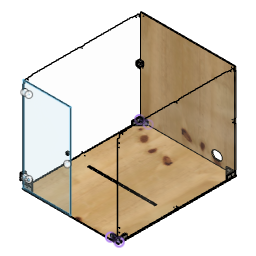
Prusa Mk3 Case (Autodesk Fusion 360 design; units mm, degrees)
Autodesk Fusion 360 part; units mm, degrees
note: some values were not read from the file. Set by a fixed rule: which sketch regions a step uses.
sketch "Sketch1" plane through (0, 0, 0) normal (0, 0, 1) x (1, 0, 0) in component "winkel"
  line L0 (0, 0) -> (42.4, 0)
  line L1 (42.4, 0) -> (42.4, 40)
  line L2 (42.4, 40) -> (0, 40)
  line L3 (0, 40) -> (0, 0)
  line L4 (2, 0) -> (2, 40)
  line L5 (4.4, 40) -> (4.4, 0)
  line L6 (7.4, 0) -> (7.4, 35)
  line L7 (7.4, 35) -> (42.4, 35)
  circle A0 centre (17.8289, 24.5711) radius 2
  line L8 (7.4, 5.6569) -> (36.7431, 35)
  line L9 (7.4, 0) -> (42.4, 35)
  line L10 (18.0066, 16.2635) -> (20.835, 13.435)
  line L11 (26.1365, 24.3934) -> (28.965, 21.565)
  line L12 (4.4, 35) -> (2, 35)
  line L13 (7.4, 35) -> (22.0716, 20.3284)
  dimension "d1" = 2.4
  dimension "d4" = 2
  dimension "d6" = 3
  dimension "d14" = 4
  dimension "d17" = 4
  dimension "d19" = 15
  dimension "d20" = 15
  dimension "d73" = 5
  dimension "d74" = 5
  dimension "d238" = 35
  dimension "d239" = 35
  dimension "d240" = 6
  constraint horizontal L0
  constraint vertical L1
  constraint horizontal L2
  constraint vertical L3
  constraint coincident L0.start L3.end
  constraint coincident L0 L4.start
  constraint perpendicular L0 L4
  constraint coincident L0 L6.start
  constraint perpendicular L0 L6
  constraint coincident L1 L7.end
  constraint perpendicular L1 L7
  constraint coincident L6 L8.start
  constraint coincident L7 L8.end
  constraint coincident L8 L10.start
  constraint coincident L9 L10.end
  constraint perpendicular L9 L10
  constraint coincident L8 L11.start
  constraint coincident L9 L11.end
  constraint perpendicular L9 L11
  constraint parallel L8 L9
  constraint coincident L2 L4.end
  constraint coincident L2 L5.start
  constraint coincident L5 L12.start
  constraint coincident L4 L12.end
  constraint perpendicular L4 L12
  constraint midpoint L8 L13.end
  constraint coincident A0.centre L13
  measures "d1" distance of L4 L5
  measures "d4" distance of L3 L4
  measures "d6" distance of L5 L6
  measures "d14" diameter of A0
  measures "d17" distance of L8 L9
  measures "d19" distance of L8.start L10
  measures "d20" distance of L8.end L11
  measures "d73" distance of L2 L7
  measures "d74" distance of L2 L12
  measures "d238" distance of L1 L6
  measures "d239" distance of L0 L7
  measures "d240" distance of A0.centre L8
extrude "Extrude1" add sketch "Sketch1" against normal blind 3 contours L0 L2 L3 L4 | L0 L4 L5 L12 | L0 L1 L2 L5 L6 L7 | L2 L4 L5 L12 | L6 L8 L9 L10 | L6 A0 L8 L13 | L8 L9 L10 L11 | L7 L8 L9 L11 | L7 A0 L8 L13 makes body 1 in component "winkel"
extrude "Extrude2" add sketch "Sketch1" along normal blind 15 contours L0 L2 L3 L4 | L0 L1 L2 L5 L6 L7 | L2 L4 L5 L12 | L6 L8 L9 L10 | L7 L8 L9 L11 bodies 1 in component "winkel"
extrude "Extrude3" add sketch "Sketch1" along normal blind 15 contours L6 L8 L9 L10 | L7 L8 L9 L11 bodies 1 in component "winkel"
chamfer "Chamfer1" distance 13 distance2 14 2 edges at (19.4208, 14.8492, 15) (27.5508, 22.9792, 15) measured on face at (26.381, 38.3333, 15) measured on face at (26.381, 38.3333, 15) on bodies 1 in component "winkel"
sketch "Sketch2" plane through (0, 40, 0) normal (0, 1, 0) x (-1, 0, 0) in component "winkel"
  line L0 (-42.4, 15) -> (-42.4, -3)
  line L1 (-42.4, -3) -> (0, -3)
  line L2 (0, -3) -> (0, 15)
  line L3 (0, 15) -> (-42.4, 15)
  circle A0 centre (-20, 7) radius 1.75
  line L4 (0, 0) -> (-42.4, 0)
  dimension "d119" = 20
  dimension "d120" = 7
  dimension "d267" = 3.5
  measures "d119" distance of L2 A0.centre
  measures "d120" distance of A0.centre L4
  measures "d267" diameter of A0
extrude "Extrude4" cut sketch "Sketch2" against normal blind 13 contours A0 bodies 1 in component "winkel"
sketch "Sketch3" plane through (0, 0, 0) normal (-1, 0, 0) x (0, -1, 0) in component "winkel"
  line L0 (-40, 15) -> (-40, -3)
  line L1 (-40, -3) -> (0, -3)
  line L2 (0, -3) -> (0, 15)
  line L3 (0, 15) -> (-40, 15)
  circle A0 centre (-20, 7) radius 1.75
  line L4 (-40, 8.75) -> (-40, 5.25)
  dimension "d264" = 20
  dimension "d265" = 7
  dimension "d266" = 3.5
  measures "d264" distance of A0.centre L4
  measures "d265" vertical distance of origin A0.centre
  measures "d266" diameter of A0
extrude "Extrude5" cut sketch "Sketch3" against normal blind 20 contours A0 bodies 1 in component "winkel"
mirror "MirrorComponent2" about plane through (0, 0, 0) normal (0, 0, 1) of bodies 1 makes body 2 in component "winkel(Mirror)"
sketch "Sketch1 (2)" plane through (0, 0, 0) normal (0, 0, 1) x (1, 0, 0) in component "grundplatte"
  line L0 (0, 0) -> (470, 0)
  line L1 (470, 0) -> (470, -580)
  line L2 (470, -580) -> (0, -580)
  line L3 (0, -580) -> (0, 0)
  circle A0 centre (18, -20) radius 1.75
  circle A1 centre (452, -20) radius 1.75
  circle A2 centre (18, -560) radius 1.75
  circle A3 centre (452, -560) radius 1.75
  circle A4 centre (16, -290) radius 1.75
  circle A5 centre (454, -290) radius 1.75
  line L4 (70, -320) -> (400, -320)
  line L5 (400, -320) -> (400, -330)
  line L6 (400, -330) -> (70, -330)
  line L7 (70, -330) -> (70, -320)
  dimension "d27" = 580
  dimension "d28" = 470
  dimension "d31" = 18
  dimension "d32" = 20
  dimension "d252" = 3.5
  dimension "d253" = 18
  dimension "d254" = 20
  dimension "d255" = 16
  dimension "d256" = 16
  dimension "d309" = 290
  dimension "d358" = 330
  dimension "d359" = 10
  dimension "d360" = 250
  dimension "d361" = 70
  constraint horizontal L0
  constraint vertical L1
  constraint horizontal L2
  constraint vertical L3
  constraint coincident L0.start L3.end
  constraint equal A0 A1
  constraint horizontal A0.centre A1.centre
  constraint equal A2 A3
  constraint equal A1 A3
  constraint vertical A1.centre A3.centre
  constraint horizontal A2.centre A3.centre
  constraint vertical A0.centre A2.centre
  constraint equal A4 A5
  constraint equal A2 A4
  constraint horizontal A4.centre A5.centre
  constraint horizontal L4
  constraint vertical L5
  constraint horizontal L6
  constraint vertical L7
  measures "d27" distance of L0.start L2.end
  measures "d28" distance of L1.end L2.end
  measures "d31" distance of L3 A0.centre
  measures "d32" distance of L0 A0.centre
  measures "d252" diameter of A0
  measures "d253" distance of L1 A1.centre
  measures "d254" distance of L2 A2.centre
  measures "d255" distance of L3 A4.centre
  measures "d256" distance of L1 A5.centre
  measures "d309" distance of L2 A4.centre
  measures "d358" distance of L5.end L6.end
  measures "d359" distance of L4.start L6.end
  measures "d360" distance of L2 L6
  measures "d361" distance of L3 L6.end
extrude "Extrude1'" add sketch "Sketch1 (2)" along normal blind 5 separate body makes body 3 in component "grundplatte"
sketch "Sketch1 (3)" plane through (0, 0, 0) normal (1, 0, 0) x (0, 1, 0) in component "seite"
  line L0 (179.5, 146.2971) -> (-400.5, 146.2971)
  line L1 (-400.5, 146.2971) -> (-400.5, 606.2971)
  line L2 (-400.5, 606.2971) -> (179.5, 606.2971)
  line L3 (179.5, 606.2971) -> (179.5, 146.2971)
  line L4 (179.5, 149.5971) -> (134.5, 149.5971)
  line L5 (134.5, 149.5971) -> (134.5, 146.2971)
  line L6 (-400.5, 149.5971) -> (-355.5, 149.5971)
  line L7 (-355.5, 149.5971) -> (-355.5, 146.2971)
  line L8 (-400.5, 164.2971) -> (-390.5, 164.2971)
  line L9 (-390.5, 164.2971) -> (-390.5, 149.5971)
  line L10 (179.5, 164.2971) -> (169.5, 164.2971)
  line L11 (169.5, 164.2971) -> (169.5, 146.2971)
  line L12 (-400.5, 588.2971) -> (-390.5, 588.2971)
  line L13 (-390.5, 588.2971) -> (-390.5, 602.9971)
  line L14 (-390.5, 602.9971) -> (-355.5, 602.9971)
  line L15 (-355.5, 602.9971) -> (-355.5, 606.2971)
  line L16 (134.5, 606.2971) -> (134.5, 602.9971)
  line L17 (134.5, 602.9971) -> (169.5, 602.9971)
  line L18 (169.5, 602.9971) -> (169.5, 588.2971)
  line L19 (169.5, 588.2971) -> (179.5, 588.2971)
  circle A0 centre (170.5, 206.2971) radius 1.75
  circle A1 centre (170.5, 186.2971) radius 1.75
  circle A2 centre (170.5, 566.2971) radius 1.75
  circle A3 centre (170.5, 546.2971) radius 1.75
  line L20 (-100, 146.2971) -> (-100, 149.5971)
  line L21 (-100, 149.5971) -> (-121, 149.5971)
  line L22 (-121, 149.5971) -> (-121, 146.2971)
  line L23 (-100, 606.2971) -> (-100, 602.9971)
  line L24 (-100, 602.9971) -> (-121, 602.9971)
  line L25 (-121, 602.9971) -> (-121, 606.2971)
  line L26 (-400.5, 386.7971) -> (-392.2, 386.7971)
  line L27 (-392.2, 386.7971) -> (-392.2, 365.7971)
  line L28 (-392.2, 365.7971) -> (-400.5, 365.7971)
  circle A4 centre (154.5, 156.2971) radius 1.75
  circle A5 centre (154.5, 596.2971) radius 1.75
  circle A6 centre (-375.5, 596.2971) radius 1.75
  circle A7 centre (-375.5, 156.2971) radius 1.75
  circle A8 centre (-385.2, 376.2971) radius 1.75
  circle A9 centre (-110.5, 156.5971) radius 1.75
  circle A10 centre (-110.5, 595.9971) radius 1.75
  dimension "d33" = 580
  dimension "d44" = 3.3
  dimension "d45" = 45
  dimension "d46" = 45
  dimension "d47" = 3.3
  dimension "d77" = 18
  dimension "d78" = 10
  dimension "d79" = 18
  dimension "d80" = 10
  dimension "d90" = 460
  dimension "d91" = 10
  dimension "d92" = 10
  dimension "d93" = 18
  dimension "d94" = 18
  dimension "d95" = 3.3
  dimension "d96" = 3.3
  dimension "d97" = 45
  dimension "d98" = 45
  dimension "d197" = 20
  dimension "d198" = 3.5
  dimension "d200" = 40
  dimension "d201" = 9
  dimension "d205" = 20
  dimension "d206" = 40
  dimension "d231" = 21
  dimension "d232" = 3.3
  dimension "d233" = 279.5
  dimension "d234" = 3.3
  dimension "d257" = 21
  dimension "d258" = 8.3
  dimension "d259" = 219.5
  dimension "d270" = 25
  dimension "d271" = 25
  dimension "d272" = 3.5
  dimension "d273" = 10
  dimension "d274" = 10
  dimension "d280" = 10.5
  dimension "d281" = 3.5
  dimension "d282" = 7
  dimension "d283" = 3.5
  dimension "d284" = 10.5
  dimension "d285" = 7
  dimension "d286" = 3.5
  dimension "d287" = 10.5
  dimension "d288" = 7
  constraint horizontal L0
  constraint vertical L1
  constraint horizontal L2
  constraint vertical L3
  constraint coincident L3 L4.start
  constraint perpendicular L3 L4
  constraint coincident L0 L5.end
  constraint perpendicular L0 L5
  constraint coincident L1 L6.start
  constraint perpendicular L1 L6
  constraint coincident L0 L7.end
  constraint perpendicular L0 L7
  constraint coincident L1 L8.start
  constraint perpendicular L1 L8
  constraint coincident L6 L9.end
  constraint perpendicular L6 L9
  constraint coincident L3 L10.start
  constraint perpendicular L3 L10
  constraint coincident L0 L11.end
  constraint perpendicular L0 L11
  constraint coincident L1 L12.start
  constraint perpendicular L1 L12
  constraint perpendicular L12 L13
  constraint perpendicular L13 L14
  constraint coincident L2 L15.end
  constraint perpendicular L2 L15
  constraint coincident L2 L16.start
  constraint perpendicular L2 L16
  constraint perpendicular L16 L17
  constraint perpendicular L17 L18
  constraint coincident L3 L19.end
  constraint perpendicular L3 L19
  constraint equal A0 A1
  constraint vertical A0.centre A1.centre
  constraint equal A2 A3
  constraint equal A0 A3
  constraint vertical A0.centre A3.centre
  constraint coincident L0 L20.start
  constraint perpendicular L0 L20
  constraint perpendicular L20 L21
  constraint coincident L0 L22.end
  constraint perpendicular L21 L22
  constraint coincident L2 L23.start
  constraint perpendicular L2 L23
  constraint perpendicular L23 L24
  constraint coincident L2 L25.end
  constraint perpendicular L2 L25
  constraint vertical L20.end L23.end
  constraint vertical L21.end L24.end
  constraint coincident L1 L26.start
  constraint perpendicular L1 L26
  constraint perpendicular L26 L27
  constraint perpendicular L27 L28
  constraint horizontal A5.centre A6.centre
  constraint vertical A6.centre A7.centre
  constraint horizontal A4.centre A7.centre
  constraint vertical A4.centre A5.centre
  constraint equal A5 A6
  constraint equal A6 A7
  constraint equal A4 A7
  measures "d33" distance of L1.end L2.end
  measures "d44" distance of L4.end L5.end
  measures "d45" distance of L4.start L4.end
  measures "d46" distance of L6.start L6.end
  measures "d47" distance of L6.end L7.end
  measures "d77" distance of L0 L8
  measures "d78" distance of L8.start L8.end
  measures "d79" distance of L0 L10
  measures "d80" distance of L10.start L10.end
  measures "d90" distance of L0.end L1.end
  measures "d91" distance of L18.end L19.end
  measures "d92" distance of L12.start L12.end
  measures "d93" distance of L2 L12.end
  measures "d94" distance of L2 L18.end
  measures "d95" distance of L16.start L16.end
  measures "d96" distance of L14.end L15.end
  measures "d97" distance of L1 L14.end
  measures "d98" distance of L3 L16.end
  measures "d197" distance of A0.centre A1.centre
  measures "d198" diameter of A0
  measures "d200" distance of L0 A1.centre
  measures "d201" distance of L3 A0.centre
  measures "d205" distance of A2.centre A3.centre
  measures "d206" distance of L2 A2.centre
  measures "d231" distance of L20.end L21.end
  measures "d232" distance of L20.start L20.end
  measures "d233" distance of L3 L20
  measures "d234" distance of L23.start L23.end
  measures "d257" distance of L26.end L27.end
  measures "d258" distance of L26.start L26.end
  measures "d259" distance of L0 L27.end
  measures "d270" distance of L3 A5.centre
  measures "d271" distance of L1 A6.centre
  measures "d272" diameter of A5
  measures "d273" distance of L2 A5.centre
  measures "d274" distance of L0 A4.centre
  measures "d280" distance of L28 A8.centre
  measures "d281" diameter of A8
  measures "d282" distance of L27 A8.centre
  measures "d283" diameter of A9
  measures "d284" distance of L22 A9.centre
  measures "d285" distance of L21 A9.centre
  measures "d286" diameter of A10
  measures "d287" distance of L25 A10.centre
  measures "d288" distance of L24 A10.centre
extrude "Extrude1''" add sketch "Sketch1 (3)" along normal blind 2 separate body contours L0 L1 L2 L3 L4 L5 L6 L7 L8 L9 L10 L11 L12 L13 L14 L15 L16 L17 L18 L19 L20 L21 L22 L23 L24 L25 L26 L27 L28 makes body 4 in component "seite"
sketch "Sketch1 (4)" plane through (0, 0, 0) normal (0, 1, 0) x (1, 0, 0) in component "hinten"
  line L0 (10.4, -408.1183) -> (471, -408.1183)
  line L1 (471, -408.1183) -> (471, 51.8817)
  line L2 (471, 51.8817) -> (10.4, 51.8817)
  line L3 (10.4, 51.8817) -> (10.4, -408.1183)
  circle A0 centre (456, 41.8817) radius 1.75
  circle A1 centre (25.4, 41.8817) radius 1.75
  circle A2 centre (456, -398.1183) radius 1.75
  circle A3 centre (25.4, -398.1183) radius 1.75
  line L4 (379, -8.1183) -> (391, -8.1183)
  arc A4 (391, -8.1183) -> (391, 31.8817) centre (391, 11.8817) ccw
  line L5 (391, 31.8817) -> (379, 31.8817)
  arc A5 (379, 31.8817) -> (379, -8.1183) centre (379, 11.8817) ccw
  line L6 (359, 11.8817) -> (411, 11.8817) construction
  circle A6 centre (21.4, -178.1183) radius 1.75
  circle A7 centre (460, -178.1183) radius 1.75
  dimension "d121" = 460
  dimension "d122" = 460.6
  dimension "d129" = 3.5
  dimension "d130" = 10
  dimension "d131" = 10
  dimension "d132" = 15
  dimension "d133" = 15
  dimension "d242" = 20
  dimension "d243" = 12
  dimension "d260" = 3.5
  dimension "d261" = 230
  dimension "d262" = 11
  dimension "d263" = 11
  dimension "d356" = 80
  dimension "d357" = 40
  constraint horizontal L0
  constraint vertical L1
  constraint horizontal L2
  constraint vertical L3
  constraint equal A1 A3
  constraint equal A0 A2
  constraint equal A2 A3
  constraint horizontal A2.centre A3.centre
  constraint vertical A0.centre A2.centre
  constraint horizontal A0.centre A1.centre
  constraint vertical A1.centre A3.centre
  constraint tangent L4 A4
  constraint tangent A4 L5
  constraint parallel L4 L5
  constraint tangent L5 A5
  constraint tangent L4 A5
  constraint midpoint A5 L6.start
  constraint midpoint A4 L6.end
  constraint horizontal L6
  constraint equal A6 A7
  constraint horizontal A6.centre A7.centre
  measures "d121" distance of L0.start L2.end
  measures "d122" distance of L0.start L0.end
  measures "d129" diameter of A3
  measures "d130" distance of L0 A2.centre
  measures "d131" distance of L2 A0.centre
  measures "d132" distance of L1 A0.centre
  measures "d133" distance of L3 A3.centre
  measures "d242" radius of A4
  measures "d243" distance of L4.start L4.end
  measures "d260" diameter of A7
  measures "d261" distance of L2 A6.centre
  measures "d262" distance of L3 A6.centre
  measures "d263" distance of L1 A7.centre
  measures "d356" distance of L1 A4.centre
  measures "d357" distance of L2 A5.centre
extrude "Extrude1'''" add sketch "Sketch1 (4)" along normal blind 5 separate body makes body 5 in component "hinten"
sketch "Sketch1 (5)" plane through (0, 0, 0) normal (0, 0, 1) x (1, 0, 0) in component "scharnier_1"
  line L0 (-72.6357, -505.4656) -> (-64.6357, -505.4656)
  line L1 (-64.6357, -505.4656) -> (-64.6357, -480.4656)
  line L2 (-64.6357, -480.4656) -> (-72.6357, -480.4656)
  line L3 (-72.6357, -480.4656) -> (-72.6357, -505.4656)
  circle A0 centre (-68.6357, -501.4656) radius 1.5
  line L4 (-72.6357, -495.4656) -> (-64.6357, -495.4656)
  dimension "d136" = 25
  dimension "d137" = 8
  dimension "d138" = 3
  dimension "d139" = 4
  dimension "d140" = 4
  dimension "d141" = 10
  constraint horizontal L0
  constraint vertical L1
  constraint horizontal L2
  constraint vertical L3
  constraint coincident L3 L4.start
  constraint coincident L1 L4.end
  constraint perpendicular L1 L4
  measures "d136" distance of L0.start L2.end
  measures "d137" distance of L1.end L2.end
  measures "d138" diameter of A0
  measures "d139" distance of L3 A0.centre
  measures "d140" distance of L0 A0.centre
  measures "d141" distance of L0 L4
extrude "Extrude1''''" add sketch "Sketch1 (5)" along normal blind 30 separate body makes body 6 in component "scharnier_1"
extrude "Extrude2'" cut sketch "Sketch1 (5)" along normal blind 20 and the other way blind -10 contours L0 L1 L3 L4 bodies 6 in component "scharnier_1"
sketch "Sketch2 (2)" plane through (-64.6357, 0, 0) normal (1, 0, 0) x (0, 1, 0) in component "scharnier_1"
  line L0 (-505.4656, 20) -> (-495.4656, 20)
  line L1 (-495.4656, 20) -> (-495.4656, 10)
  line L2 (-495.4656, 10) -> (-505.4656, 10)
  line L3 (-505.4656, 10) -> (-505.4656, 0)
  line L4 (-505.4656, 0) -> (-480.4656, 0)
  line L5 (-480.4656, 0) -> (-480.4656, 30)
  line L6 (-480.4656, 30) -> (-505.4656, 30)
  line L7 (-505.4656, 30) -> (-505.4656, 20)
  circle A0 centre (-488.4656, 5) radius 1.75
  circle A1 centre (-488.4656, 25) radius 1.75
  circle A2 centre (-488.4656, 25) radius 3
  circle A3 centre (-488.4656, 5) radius 3
  dimension "d180" = 3.5
  dimension "d202" = 8
  dimension "d203" = 5
  dimension "d204" = 20
  dimension "d213" = 6
  constraint equal A0 A1
  constraint vertical A0.centre A1.centre
  constraint concentric A1 A2
  constraint concentric A0 A3
  constraint equal A2 A3
  measures "d180" diameter of A1
  measures "d202" distance of L5 A1.centre
  measures "d203" distance of L6 A1.centre
  measures "d204" distance of A0.centre A1.centre
  measures "d213" diameter of A3
extrude "Extrude3'" cut sketch "Sketch2 (2)" against normal blind 30 contours A0 | A1 bodies 6 in component "scharnier_1"
fillet "Fillet1" radius 3 5 edges at (-64.6357, -505.4656, 25) (-64.6357, -505.4656, 5) (-72.6357, -505.4656, 5) (-72.6357, -505.4656, 25) (-72.6357, -495.4656, 15) on bodies 6 in component "scharnier_1"
chamfer "Chamfer1'" distance 6 distance2 12.5 1 edges at (-72.6357, -480.4656, 15) measured on face at (-67.3024, -480.4656, 10) on bodies 6 in component "scharnier_1"
extrude "Extrude4'" cut sketch "Sketch2 (2)" along normal blind -4 and the other way blind 8 contours A2 | A3 bodies 6 in component "scharnier_1"
sketch "Sketch1 (6)" plane through (0, 0, 0) normal (0, 0, 1) x (1, 0, 0) in component "scharnier_2"
  line L0 (36, -516) -> (36, -526)
  line L1 (36, -526) -> (-4, -526)
  line L2 (-4, -526) -> (-4, -518)
  circle A0 centre (0, -522) radius 1.5
  line L3 (8, -516) -> (36, -516)
  line L4 (3, -518) -> (3, -519)
  line L5 (3, -519) -> (8, -519)
  line L6 (36, -521) -> (2.8865, -526)
  line L7 (8, -519) -> (8, -516)
  line L8 (-4, -518) -> (3, -518)
  dimension "d154" = 8
  dimension "d155" = 4
  dimension "d156" = 4
  dimension "d158" = 3
  dimension "d159" = 2
  dimension "d181" = 7
  dimension "d182" = 1
  dimension "d183" = 40
  dimension "d184" = 5
  constraint horizontal L8
  constraint vertical L0
  constraint horizontal L1
  constraint vertical L2
  constraint perpendicular L4 L8
  constraint perpendicular L4 L5
  constraint midpoint L0 L6.start
  constraint coincident L1 L6.end
  constraint vertical L7
  measures "d154" distance of L2.end L1.end
  measures "d155" distance of L1 A0.centre
  measures "d156" distance of L2 A0.centre
  measures "d158" diameter of A0
  measures "d159" distance of L3 L8
  measures "d181" distance of L2.end L4.start
  measures "d182" distance of L4.start L4.end
  measures "d183" distance of L0 L2
  measures "d184" distance of L4.end L5.end
extrude "Extrude1'''''" add sketch "Sketch1 (6)" along normal blind 9.75 separate body contours L0 L1 L2 L3 L4 L5 L6 L7 L8 makes body 7 in component "scharnier_2"
fillet "Fillet1'" radius 2.5 4 edges at (-4, -526, 4.875) (-4, -518, 4.875) (36, -521, 4.875) (3, -518, 4.875) on bodies 7 in component "scharnier_2"
sketch "Sketch2 (3)" plane through (0, -516, 0) normal (0, 1, 0) x (-1, 0, 0) in component "scharnier_2"
  line L0 (-36, 0) -> (-8, 0)
  line L1 (-8, 0) -> (-8, 9.75)
  line L2 (-8, 9.75) -> (-36, 9.75)
  line L3 (-36, 9.75) -> (-36, 0)
  circle A0 centre (-32, 4.875) radius 1.75
  circle A1 centre (-12, 4.875) radius 1.75
  circle A2 centre (-12, 4.875) radius 3
  circle A3 centre (-32, 4.875) radius 3
  dimension "d186" = 3.5
  dimension "d187" = 20
  dimension "d188" = 4.875
  dimension "d189" = 4
  dimension "d192" = 6
  constraint equal A0 A1
  constraint horizontal A0.centre A1.centre
  constraint concentric A1 A2
  constraint concentric A0 A3
  constraint equal A2 A3
  measures "d186" diameter of A0
  measures "d187" distance of A0.centre A1.centre
  measures "d188" distance of L2 A0.centre
  measures "d189" distance of L1 A1.centre
  measures "d192" diameter of A2
extrude "Extrude2''" cut sketch "Sketch2 (3)" against normal blind 15 contours A0 | A1 bodies 7 in component "scharnier_2"
extrude "Extrude3''" cut sketch "Sketch2 (3)" along normal blind -11 and the other way blind 5 contours A3 bodies 7 in component "scharnier_2"
fillet "Fillet2" radius 2 2 edges at (8, -519, 4.875) (3, -519, 4.875) on bodies 7 in component "scharnier_2"
extrude "Extrude4''" cut sketch "Sketch2 (3)" along normal blind -13 and the other way blind 8 contours A2 bodies 7 in component "scharnier_2"
sketch "Sketch1 (7)" plane through (0, 0, 0) normal (0, 1, 0) x (1, 0, 0) in component "tür"
  line L0 (-305, -450) -> (-75.2, -450)
  line L1 (-75.2, -450) -> (-75.2, 8)
  line L2 (-75.2, 8) -> (-305, 8)
  line L3 (-305, 8) -> (-305, -450)
  circle A0 centre (-299.2, -41) radius 1.75
  circle A1 centre (-279.2, -41) radius 1.75
  circle A2 centre (-299.2, -401) radius 1.75
  circle A3 centre (-279.2, -401) radius 1.75
  circle A4 centre (-90.2, -201) radius 1.75
  dimension "d168" = 458
  dimension "d169" = 229.8
  dimension "d207" = 20
  dimension "d208" = 3.5
  dimension "d209" = 5.8
  dimension "d210" = 49
  dimension "d218" = 49
  dimension "d296" = 3.5
  dimension "d297" = 15
  constraint horizontal L0
  constraint vertical L1
  constraint horizontal L2
  constraint vertical L3
  constraint equal A0 A1
  constraint horizontal A0.centre A1.centre
  constraint horizontal A2.centre A3.centre
  constraint vertical A0.centre A2.centre
  constraint vertical A1.centre A3.centre
  constraint equal A2 A3
  constraint equal A0 A2
  measures "d168" distance of L0.start L2.end
  measures "d169" distance of L1.end L2.end
  measures "d207" distance of A0.centre A1.centre
  measures "d208" diameter of A0
  measures "d209" distance of L3 A0.centre
  measures "d210" distance of L2 A0.centre
  measures "d218" distance of L0 A3.centre
  measures "d296" diameter of A4
  measures "d297" distance of L1 A4.centre
extrude "Extrude1''''''" add sketch "Sketch1 (7)" along normal blind 2 separate body contours L0 L1 L2 L3 | A4 makes body 8 in component "tür"
sketch "Sketch1 (8)" plane through (0, 0, 0) normal (0, 0, 1) x (1, 0, 0) in component "WInkel2"
  line L0 (-50.6004, -235) -> (-30, -235)
  line L1 (-30, -235) -> (-30, -255)
  line L2 (-30, -255) -> (-50.6004, -255)
  line L3 (-50.6004, -255) -> (-50.6004, -235)
  line L4 (-48.1004, -235) -> (-48.1004, -255)
  line L5 (-45.9004, -235) -> (-45.9004, -255)
  line L6 (-42.9004, -235) -> (-42.9004, -255)
  line L7 (-42.9004, -238) -> (-30, -238)
  line L8 (-42.9004, -252) -> (-30, -252)
  circle A0 centre (-35, -245) radius 1.75
  dimension "d219" = 2.2
  dimension "d220" = 2.5
  dimension "d221" = 3
  dimension "d222" = 3
  dimension "d223" = 3
  dimension "d224" = 20
  dimension "d289" = 3.5
  constraint horizontal L0
  constraint vertical L1
  constraint horizontal L2
  constraint vertical L3
  constraint coincident L0 L4.start
  constraint coincident L2 L4.end
  constraint perpendicular L2 L4
  constraint coincident L0 L5.start
  constraint coincident L2 L5.end
  constraint perpendicular L2 L5
  constraint coincident L0 L6.start
  constraint coincident L2 L6.end
  constraint perpendicular L2 L6
  constraint coincident L6 L7.start
  constraint coincident L1 L7.end
  constraint perpendicular L1 L7
  constraint coincident L6 L8.start
  constraint coincident L1 L8.end
  constraint perpendicular L1 L8
  measures "d219" distance of L4 L5
  measures "d220" distance of L3 L4
  measures "d221" distance of L5 L6
  measures "d222" distance of L2 L8
  measures "d223" distance of L0 L7
  measures "d224" distance of L0.start L2.end
  measures "d289" diameter of A0
extrude "Extrude1'''''''" add sketch "Sketch1 (8)" against normal blind 3 separate body makes body 9 in component "WInkel2"
extrude "Extrude2'''" add sketch "Sketch1 (8)" along normal blind 15 contours L0 L2 L3 L4 | L0 L2 L5 L6 | L0 L1 L6 L7 | L1 L2 L6 L8 bodies 9 in component "WInkel2"
chamfer "Chamfer1''" distance 12 distance2 10 2 edges at (-30, -236.5, 15) (-30, -253.5, 15) measured on face at (-44.9004, -242.6667, 15) measured on face at (-44.9004, -242.6667, 15) on bodies 9 in component "WInkel2"
sketch "Sketch2 (4)" plane through (-50.6004, 0, 0) normal (-1, 0, 0) x (0, -1, 0) in component "WInkel2"
  line L0 (235, 15) -> (235, -3)
  line L1 (235, -3) -> (255, -3)
  line L2 (255, -3) -> (255, 15)
  line L3 (255, 15) -> (235, 15)
  circle A0 centre (245, 7) radius 1.75
  line L4 (235, 0) -> (255, 0)
  dimension "d275" = 10
  dimension "d276" = 7
  dimension "d277" = 3.5
  measures "d275" distance of L0 A0.centre
  measures "d276" distance of A0.centre L4
  measures "d277" diameter of A0
extrude "Extrude3'''" cut sketch "Sketch2 (4)" against normal blind 30 contours A0 bodies 9 in component "WInkel2"
sketch "Sketch1 (9)" plane through (0, 0, 0) normal (0, 1, 0) x (1, 0, 0) in component "türnupsi"
  line L0 (-3.65, -1.0015) -> (-3.65, 2.9985)
  line L1 (-3.65, 2.9985) -> (-7.65, 4.9985)
  line L2 (-7.65, 4.9985) -> (-7.65, 11.9985)
  line L3 (-7.65, 11.9985) -> (-4.2801, 13.9985)
  line L4 (-4.2801, 13.9985) -> (-1.65, 13.9985)
  line L5 (-1.65, 13.9985) -> (-1.65, -1.0015)
  line L6 (-1.65, -1.0015) -> (-3.65, -1.0015)
  dimension "d298" = 1.65
  dimension "d299" = 2
  dimension "d300" = 4
  dimension "d301" = 7
  dimension "d302" = 2
  dimension "d303" = 6
  dimension "d304" = 15
  constraint vertical L0
  constraint parallel L0 L2
  constraint horizontal L4
  constraint perpendicular L4 L5
  constraint perpendicular L0 L6
  measures "d298" distance of origin L5
  measures "d299" distance of L0 L5
  measures "d300" distance of L0.start L0.end
  measures "d301" distance of L1.end L2.end
  measures "d302" vertical distance of L2.end L3.end
  measures "d303" distance of L2 L5
  measures "d304" distance of L4.end L5.end
revolve "Revolve1" add sketch "Sketch1 (9)" angle 360 about axis through (0, 0, 1.75) along (0, 0, 1) separate body makes body 10 in component "türnupsi"
fillet "Fillet1''" radius 1 3 edges at (-7.1323, 2.7664, -4.9985) (-7.1323, 2.7664, -11.9985) (-3.9904, 1.5477, -13.9985) on bodies 10 in component "türnupsi"
chamfer "Chamfer1'''" distance 2 angle 45 1 edges at (-1.5383, 0.5967, -13.9985) on bodies 10 in component "türnupsi"
move_body "Move1" bodies 10 to x (0, 0, 1) y (1, 0, 0) z (0, 1, 0) at (235.9709, -596.0015, 191.7935) in component "türnupsi"
component "winkel" placed x (1, 0, 0) y (0, 1, 0) z (0, 0, 1) at (21.5107, -79.2529, -54.9092)
component "winkel" placed x (-1, 0, 0) y (0, -1, 0) z (0, 0, 1) at (491.5107, -569.2529, -54.9092)
component "winkel(Mirror)" placed x (1, 0, 0) y (0, -1, 0) z (0, 0, -1) at (21.5107, -569.2529, -54.9092)
component "winkel(Mirror)" placed x (-1, 0, 0) y (0, 1, 0) z (0, 0, -1) at (491.5107, -79.2529, -54.9092)
component "grundplatte" placed x (1, 0, 0) y (0, 1, 0) z (0, 0, 1) at (21.5107, -34.2529, -62.9092)
component "seite" placed x (-1, 0, 0) y (0, -1, 0) z (0, 0, 1) at (26.0107, -434.7529, -204.5063)
component "seite" placed x (-1, 0, 0) y (0, -1, 0) z (0, 0, 1) at (489.0107, -434.7529, -204.5063)
component "hinten" placed x (1, 0, 0) y (0, 1, 0) z (0, 0, 1) at (15.8107, -39.2529, -6.0275)
component "scharnier_1" placed x (1, 0, 0) y (0, 1, 0) z (0, 0, 1) at (88.6465, -116.7873, -23.2092)
component "scharnier_2" placed x (1, 0, 0) y (0, 1, 0) z (0, 0, 1) at (20.0107, -96.2529, -12.9592)
component "tür" placed x (1, 0, 0) y (0, 1, 0) z (0, 0, 1) at (331.2107, -612.2529, -49.0842)
component "WInkel2" placed x (1, 0, 0) y (0, 1, 0) z (0, 0, 1) at (72.6325, -69.2961, -54.8413)
component "WInkel2" placed x (1, 0, 0) y (0, 0, 1) z (0, -1, 0) at (72.1756, -42.566, 436.733)
component "türnupsi" placed x (1, 0, 0) y (0, 1, 0) z (0, 0, 1) at (0, 0, 0)
equation "breite_aussen = 470 mm"
equation "tiefe_aussen = 580 mm"
equation "d27 = tiefe_aussen"
equation "d28 = breite_aussen"
equation "d33 = tiefe_aussen"
equation "d44 = d95"
equation "d45 = d98"
equation "d46 = d98"
equation "d47 = d95"
equation "d77 = d79"
equation "höhe_innen = 460 mm"
equation "d90 = höhe_innen"
equation "d93 = d94"
equation "d94 = d79"
equation "d96 = d95"
equation "d97 = d98"
equation "d121 = höhe_innen"
equation "d122 = breite_aussen - ( 2 * 2.5 ) * 1 mm - ( 2 * 2.2 ) * 1 mm"
equation "d126 = -2.2 mm - 2.5 mm"
equation "d130 = d131"
equation "d132 = d133"
equation "d139 = d137 / 2"
equation "d155 = d154 / 2"
equation "d168 = höhe_innen - 2 mm"
equation "d169 = ( breite_aussen - ( 2 * 2.5 ) * 1 mm - ( 2 * 2.2 ) * 1 mm - 1 mm ) / 2"
equation "d188 = ( 9.75 / 2 ) * 1 mm"
equation "d206 = d200"
equation "d232 = d47"
equation "d233 = ( d33 - d231 ) / 2"
equation "d234 = d95"
equation "d256 = d255"
equation "d259 = ( d90 - d257 ) / 2"
equation "d261 = d121 / 2"
equation "d263 = d262"
equation "d274 = d273"
equation "d280 = d257 / 2"
equation "d284 = d231 / 2"
equation "d287 = ( 21 / 2 ) * 1 mm"
equation "d309 = d27 / 2"
equation "d361 = ( d28 - d358 ) / 2"
